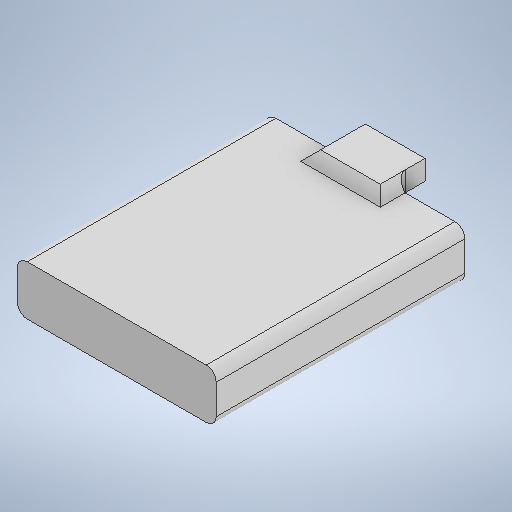
# Autodesk Inventor part: Batterie
Saved by Autodesk Inventor 2025.2 (Build 292293000, 293)
## iProperties
Created: 2024-11-18
Part Number: Batterie
Material: Generisch
Document SubType Name: Modeling
Designer: tills
Density: 1 g/cm^3
Appearance: Vorgabe
Author: tills
Autodesk Inventor part; units mm, degrees
ref_plane "YZ Plane" through (0, 0, 0) normal (1, 0, 0) x (0, 1, 0)
ref_plane "XZ Plane" through (0, 0, 0) normal (0, 1, 0) x (-1, 0, 0)
ref_plane "XY Plane" through (0, 0, 0) normal (0, 0, 1) x (1, 0, 0)
sketch "Skizze1" plane through (0, 0, 0) normal (0, 1, 0) x (-1, 0, 0)
  line L0 (10, 12.5) -> (-10, 12.5)
  line L1 (-10, 12.5) -> (-10, -12.5)
  line L2 (-10, -12.5) -> (10, -12.5)
  line L3 (10, -12.5) -> (10, 12.5)
  line L4 (10, 12.5) -> (-10, -12.5) construction
  line L5 (-10, 12.5) -> (10, -12.5) construction
  point P0 (0, 0)
  dimension "d0" = 20
  dimension "d1" = 25
  constraints: 12 end point, 2 midpoint, 2 parallel, 1 horizontal, 1 perpendicular
  measures "d0" distance of L1.end L2.end
  measures "d1" distance of L0.end L1.end
extrude "Extrusion1" add sketch "Skizze1" along normal blind 5
fillet "Rundung1" radius 1 4 edges at (-10, 5, 0) (-10, 0, 0) (10, 5, 0) (10, 0, 0)
sketch "Skizze2" plane through (9, 0, -12.5) normal (0, 0, -1) x (-1, 0, 0)
  line L0 (0, 5) -> (18, 5) projected
  line L1 (6, 4) -> (12, 4)
  line L2 (12, 4) -> (12, 6)
  line L3 (12, 6) -> (6, 6)
  line L4 (6, 6) -> (6, 4)
  line L5 (6, 4) -> (12, 6) construction
  line L6 (12, 4) -> (6, 6) construction
  point P0 (9, 0)
  point P1 (9, 5)
  dimension "d5" = 2
  dimension "d6" = 6
  constraints: 12 end point, 3 midpoint, 2 parallel, 1 horizontal, 1 perpendicular
  measures "d5" distance of L1.end L2.end
  measures "d6" distance of L2.end L3.end
extrude "Extrusion2" add sketch "Skizze2" along normal blind 3 and the other way blind 1.5
chamfer "Fasen1" distance 1 angle 45 1 edges at (0, 5, -11)
chamfer "Fasen2" distance 1 angle 45 2 edges at (-3, 5, -10.5) (-3, 5, -11.75)
chamfer "Fasen3" distance 1 angle 45 2 edges at (3, 5, -10.5001) (3, 5, -11.75)
fillet "Rundung2" radius 1 5 edges at (3, 5.5, -12.5) (3, 4.5, -12.5) (0, 4, -12.5) (-3, 4.5, -12.5) (-3, 5.5, -12.5)
